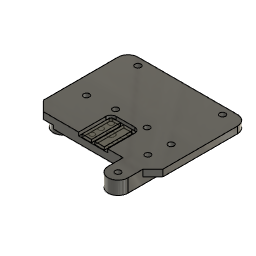
Top Plate Mjølnir (Autodesk Fusion 360 design; units mm, degrees)
Autodesk Fusion 360 part; units mm, degrees
ref_plane "WorkPlane1" through (21, -14, 35) normal (0, 0, 1) x (1, 0, 0)
sketch "Sketch2" plane through (0, 24.7, 35) normal (0, 0, 1) x (1, 0, 0)
  circle A0 centre (0, -50.925) radius 2.25
  line L0 (0, -35.7) -> (0, -50.925) construction
  line L1 (-6, -50.925) -> (6, -50.925) construction
  circle A1 centre (0, -50.925) radius 11 construction
  line L2 (18, -7.7) -> (-18, -7.7) construction
  line L3 (-30, -4.7) -> (-30, -13.7) construction
  line L4 (30, -13.7) -> (30, -4.7) construction
  circle A2 centre (-25.5, -40.2) radius 1.75 construction
  circle A3 centre (25.5, -40.2) radius 1.75 construction
  line L5 (-30, -35.7) -> (-30, -44.7) construction
  line L6 (-18, -41.7) -> (-13, -41.7) construction
  line L7 (30, -44.7) -> (30, -35.7) construction
  circle A4 centre (-25.5, -9.2) radius 1.75
  circle A5 centre (25.5, -9.2) radius 1.75
  circle A6 centre (25.5, -40.2) radius 1.75
  circle A7 centre (-25.5, -40.2) radius 1.75
  line L8 (-18, -7.7) -> (22, -7.7) construction
  line L9 (-30, -44.7) -> (-21, -44.7) construction
  line L10 (21, -44.7) -> (30, -44.7) construction
  line L11 (-30, -4.7) -> (30, -4.7)
  line L12 (30, -4.7) -> (30, -61.7)
  line L13 (30, -61.7) -> (-30, -61.7)
  line L14 (-30, -61.7) -> (-30, -4.7)
  circle A8 centre (25.5, -9.2) radius 1.75
  circle A9 centre (-25.5, -9.2) radius 1.75
  line L15 (30, -4.7) -> (21, -4.7)
  line L16 (-21, -4.7) -> (-30, -4.7)
  line L17 (-30, -13.7) -> (30, -13.7)
  line L18 (-13, -35.7) -> (-30, -35.7)
  line L19 (21, -4.7) -> (18, -7.7)
  line L20 (-18, -7.7) -> (-21, -4.7)
  line L21 (-21, -44.7) -> (-18, -41.7)
  line L22 (18, -41.7) -> (21, -44.7)
  line L23 (-30, -4.7) -> (-36, -4.7)
  line L24 (-36, -4.7) -> (-36, -61.7)
  line L25 (-36, -61.7) -> (-30, -61.7)
  line L26 (-30, -61.7) -> (-30, -4.7)
  line L27 (30, -4.7) -> (36, -4.7)
  line L28 (36, -4.7) -> (36, -61.7)
  line L29 (36, -61.7) -> (30, -61.7)
  line L30 (30, -61.7) -> (30, -4.7)
  line L31 (13, -35.7) -> (13, -41.7)
  line L32 (13, -41.7) -> (18, -41.7)
  line L33 (30, -35.7) -> (13, -35.7)
  line L34 (-13, -35.7) -> (13, -35.7)
  line L35 (-13, -41.7) -> (-13, -35.7)
  dimension "d5288" = 12
  dimension "d6330" = 4.5
  dimension "d6343" = 22
  dimension "d8089" = 10.725
  dimension "d8579" = 3.5
  dimension "d8774" = 72
  dimension "d9194" = 57
  constraint coincident A0.centre L0.end
  constraint horizontal L1
  constraint midpoint A0.centre L1
  constraint concentric A0 A1
  constraint vertical L0
  constraint coincident L2.end L8.start
  constraint concentric A4 A9
  constraint concentric A5 A8
  constraint concentric A3 A6
  constraint concentric A2 A7
  constraint equal A4 A5
  constraint equal A5 A6
  constraint equal A6 A7
  constraint horizontal L8
  constraint horizontal L11
  constraint vertical L12
  constraint horizontal L13
  constraint vertical L14
  constraint coincident L5.start L14
  constraint coincident L4.start L12
  constraint coincident L4.end L11
  constraint horizontal L23
  constraint vertical L24
  constraint horizontal L25
  constraint vertical L26
  constraint coincident L3.start L11.start
  constraint coincident L13.end L14.start
  constraint symmetric L0 L3.start L4.end
  constraint symmetric L0 L23.end L27.end
  constraint symmetric L0 L24.end L28.end
  constraint symmetric L0 L13.end L12.end
  constraint midpoint L0.start L34
  measures "d5288" distance of L1.start L1.end
  measures "d6330" diameter of A0
  measures "d6343" diameter of A1
  measures "d8089" vertical distance of A0.centre A3.centre
  measures "d8579" diameter of A4
  measures "d8774" distance of L24 L28
  measures "d9194" distance of L23.end L24.end
extrude "Extrude2" add sketch "Sketch2" along normal blind 4 makes body 1
sketch "Sketch16" plane through (0, 0, 39) normal (0, 0, 1) x (-1, 0, 0)
  circle A0 centre (0, 26.225) radius 8 construction
  line L0 (-5.6569, 20.5681) -> (5.6569, 20.5681)
  line L1 (5.6569, 20.5681) -> (5.6569, 31.8819)
  line L2 (5.6569, 31.8819) -> (-5.6569, 31.8819)
  line L3 (-5.6569, 31.8819) -> (-5.6569, 20.5681)
  line L4 (-5.6569, 20.5681) -> (5.6569, 31.8819) construction
  line L5 (5.6569, 20.5681) -> (-5.6569, 31.8819) construction
  circle A1 centre (0, 26.225) radius 2.25
  line L6 (36, 37) -> (-36, 37)
  line L7 (-36, -20) -> (36, -20)
  circle A2 centre (25.5, 15.5) radius 1.75
  circle A3 centre (25.5, -15.5) radius 1.75
  line L8 (36, -20) -> (36, 37)
  line L9 (-36, 37) -> (-36, -20)
  circle A4 centre (-25.5, -15.5) radius 1.75
  circle A5 centre (-25.5, 15.5) radius 1.75
  point P0 (0, 26.225)
  dimension "d8592" = 16
  constraint horizontal L0
  constraint perpendicular L0 L1
  constraint parallel L0 L2
  constraint parallel L1 L3
  constraint coincident A0 L0.start
  constraint coincident L4 P0
  constraint coincident L5 P0
  constraint equal L0 L3
  constraint coincident P0 A0.centre
  measures "d8592" diameter of A0
hole "Hole8" at (-5.6569, -20.5681, 39) at (-5.6569, -31.8819, 39) at (5.6569, -20.5681, 39) at (5.6569, -31.8819, 39) direction (0, 0, -1) diameter 2.9 depth 7 tip angle 118 bodies 1
hole "Hole1" at (-6, -26.225, 35) at (6, -26.225, 35) direction (0, 0, 1) diameter 2.9 depth 10 tip angle 180 bodies 1
sketch "Sketch18" plane through (0, 0, 35) normal (0, 0, -1) x (1, 0, 0)
  circle A0 centre (-25.5, -15.5) radius 1.75
  circle A1 centre (0, 26.225) radius 2.25
  circle A2 centre (-25.5, 15.5) radius 1.75
  line L0 (-36, -20) -> (36, -20)
  line L1 (36, -20) -> (36, 37)
  line L2 (36, 37) -> (-36, 37)
  line L3 (-36, 37) -> (-36, -20)
  line L4 (-19.5, 26.225) -> (17.5, 26.225) construction
  line L5 (-1, 26.225) -> (-1, 23.941) construction
  line L6 (0, 26.225) -> (0, 14.975) construction
  line L7 (0, 14.975) -> (10, 14.975) construction
  circle A3 centre (10, 14.975) radius 3
  circle A4 centre (-6, 26.225) radius 1.45
  circle A5 centre (6, 26.225) radius 1.45
  line L8 (-9.5, 24) -> (9.5, 24) construction
  line L9 (9.5, 24) -> (9.5, 14) construction
  line L10 (9.5, 14) -> (-9.5, 14) construction
  line L11 (-9.5, 14) -> (-9.5, 24) construction
  line L12 (0, 24) -> (0, 26.225) construction
  circle A6 centre (9.5, 24) radius 1.6 construction
  circle A7 centre (25.5, -15.5) radius 1.75
  circle A8 centre (25.5, 15.5) radius 1.75
  arc A9 (-13, 17) -> (13, 17) centre (0, 43.6667) ccw construction
  line L13 (13, 17) -> (13, 11) construction
  line L14 (13, 11) -> (-13, 11) construction
  circle A10 centre (5.6569, 20.5681) radius 1.45
  circle A11 centre (-5.6569, 20.5681) radius 1.45
  circle A12 centre (-5.6569, 31.8819) radius 1.45
  circle A13 centre (5.6569, 31.8819) radius 1.45
  line L15 (-13, 11) -> (-13, 17)
  point P0 (-10, 14.975)
  dimension "d8760" = 37
  dimension "d8761" = 1
  dimension "d8762" = 90
  dimension "d8763" = 10
  dimension "d8764" = 6
  dimension "d8765" = 11.25
  dimension "d8769" = 19
  dimension "d8770" = 10
  dimension "d8771" = 2.225
  dimension "d8772" = 3.2
  constraint horizontal L4
  constraint coincident A1.centre L4
  constraint midpoint L4 L5.start
  constraint perpendicular L4 L5
  constraint coincident A1.centre L6.start
  constraint perpendicular L4 L6
  constraint coincident L7.end A3.centre
  constraint symmetric L6 L7.end P0
  constraint horizontal L8
  constraint vertical L9
  constraint horizontal L10
  constraint vertical L11
  constraint midpoint L8 L12.start
  constraint perpendicular L8 L12
  constraint coincident L8.end L9.start
  measures "d8760" distance of L4.start L4.end
  measures "d8761" distance of A1.centre L5
  measures "d8762" angle of L6 L7
  measures "d8763" distance of L6.end L7.end
  measures "d8764" diameter of A3
  measures "d8765" distance of A1.centre L6.end
  measures "d8769" distance of L8.start L8.end
  measures "d8770" distance of L8.start L10.end
  measures "d8771" vertical distance of A1.centre L8.end
  measures "d8772" diameter of A6
hole "Hole11" at (9.5, -14, 35) at (-9.5, -14, 35) direction (0, 0, 1) diameter 3.4 depth 11 tip angle 118 bodies 1
chamfer "Chamfer8" distance 6 angle 45 2 edges at (-36, -37, 37) (36, -37, 37) on bodies 1
sketch "Sketch20" plane through (0, 0, 39) normal (0, 0, 1) x (-1, 0, 0)
  circle A0 centre (-9.5, 14) radius 1.7
  circle A1 centre (6, 26.225) radius 1.45
  circle A2 centre (-6, 26.225) radius 1.45
  circle A3 centre (0, 26.225) radius 2.25
  circle A4 centre (25.5, -15.5) radius 1.75
  line L0 (-36, -20) -> (36, -20)
  line L1 (36, -20) -> (36, 31)
  line L2 (30, 37) -> (-30, 37)
  line L3 (-36, 31) -> (-36, -20)
  line L4 (0, 37) -> (0, 53.2929) construction
  line L5 (-30, 37) -> (-36, 31)
  line L6 (36, 31) -> (30, 37)
  line L7 (30, 37) -> (18, 37)
  line L8 (18, 37) -> (18, 52)
  line L9 (18, 52) -> (30, 52)
  line L10 (30, 52) -> (30, 37)
  line L11 (-30, 52) -> (-30, 37)
  line L12 (-30, 37) -> (-18, 37)
  line L13 (-18, 37) -> (-18, 52)
  line L14 (-18, 52) -> (-30, 52)
  circle A5 centre (9.5, 14) radius 1.7
  circle A6 centre (-25.5, -15.5) radius 1.75
  circle A7 centre (25.5, 15.5) radius 1.75
  circle A8 centre (-25.5, 15.5) radius 1.75
  line L15 (30, 37) -> (18, 37)
  line L16 (18, 37) -> (18, 20)
  line L17 (18, 20) -> (30, 20)
  line L18 (30, 20) -> (30, 37)
  line L19 (-18, 37) -> (-18, 20)
  line L20 (-18, 20) -> (-30, 20)
  line L21 (-30, 37) -> (-18, 37)
  line L22 (-30, 20) -> (-30, 37)
  circle A9 centre (-5.6569, 20.5681) radius 1.45
  circle A10 centre (5.6569, 20.5681) radius 1.45
  circle A11 centre (5.6569, 31.8819) radius 1.45
  circle A12 centre (-5.6569, 31.8819) radius 1.45
  dimension "d9257" = 12
  dimension "d9258" = 15
  dimension "d9259" = 36
  dimension "d9371" = 17
  constraint midpoint L2 L4.start
  constraint perpendicular L2 L4
  constraint horizontal L7
  constraint vertical L8
  constraint horizontal L9
  constraint vertical L10
  constraint coincident L2.start L6.end
  constraint symmetric L4 L2.start L2.end
  constraint symmetric L4 L7.end L12.end
  constraint symmetric L4 L8.end L13.end
  constraint symmetric L4 L9.end L11.start
  constraint horizontal L15
  constraint vertical L16
  constraint horizontal L17
  constraint vertical L18
  constraint coincident L8 L7.end
  constraint symmetric L4 L16.end L19.end
  constraint symmetric L4 L17.end L20.end
  measures "d9257" distance of L2.start L7.end
  measures "d9258" distance of L2.start L9.end
  measures "d9259" distance of L8 L13
  measures "d9371" distance of L2.start L17.end
extrude "Extrude17" add sketch "Sketch20" against normal blind 8 contours L2 L11 L12 L13 L14 L21 | L2 L12 L19 L20 L21 L22 | L2 L7 L15 L16 L17 L18 bodies 1
sketch "Sketch22" plane through (0, 0, 31) normal (0, 0, -1) x (1, 0, 0)
  circle A0 centre (24, 46) radius 1.5 construction
  line L0 (24, 46) -> (24, 28) construction
  line L1 (30, 52) -> (18, 52)
  line L2 (18, 52) -> (18, 20)
  line L3 (30, 20) -> (30, 52)
  line L4 (24, 52) -> (24, 46) construction
  circle A1 centre (24, 46) radius 6
  line L5 (-30, 37) -> (-30, 20)
  line L6 (-30, 20) -> (-18, 20)
  line L7 (-18, 20) -> (-18, 37)
  line L8 (-18, 37) -> (-30, 37)
  line L9 (-30, 37) -> (-30, 20)
  line L10 (-30, 20) -> (-18, 20)
  line L11 (-18, 20) -> (-18, 37)
  line L12 (-18, 37) -> (-30, 37)
  line L13 (18, 20) -> (30, 20)
  line L14 (-18, 37) -> (18, 37)
  dimension "d9221" = 18
  dimension "d9372" = 3
  constraint coincident A0.centre L0.start
  constraint vertical L0
  constraint concentric A0 A1
  constraint tangent L3 A1
  constraint vertical L4
  constraint midpoint L1 L4.start
  constraint tangent L1 A1
  measures "d9221" distance of A0.centre L0.end
  measures "d9372" diameter of A0
fillet "Fillet9" radius 6 4 edges at (30, -52, 35) (18, -52, 35) (-18, -37, 33) (-30, -37, 33) on bodies 1
hole "Hole16" at (24, -46, 31) at (24, -28, 31) direction (0, 0, 1) diameter 3.4 depth 70 tip angle 180 bodies 1
chamfer "Chamfer9" distance 3 angle 45 2 edges at (-18, -20, 33) (18, -20, 33) on bodies 1
fillet "Fillet10" radius 6 2 edges at (36, 20, 37) (-36, 20, 37) on bodies 1
sketch "Sketch25" plane through (0, 0, 35) normal (0, 0, -1) x (1, 0, 0)
  circle A0 centre (25.5, -15.5) radius 1.75
  circle A1 centre (-25.5, -15.5) radius 1.75
  circle A2 centre (25.5, 15.5) radius 1.75
  circle A3 centre (0, 26.225) radius 2.25
  circle A4 centre (-25.5, 15.5) radius 1.75
  circle A5 centre (5.6569, 31.8819) radius 1.45
  circle A6 centre (-5.6569, 31.8819) radius 1.45
  circle A7 centre (-5.6569, 20.5681) radius 1.45
  circle A8 centre (5.6569, 20.5681) radius 1.45
  circle A9 centre (6, 26.225) radius 1.45
  circle A10 centre (-6, 26.225) radius 1.45
  circle A11 centre (-9.5, 14) radius 1.7
  circle A12 centre (9.5, 14) radius 1.7
  arc A13 (-36, -14) -> (-30, -20) centre (-30, -14) ccw
  line L0 (-30, -20) -> (30, -20)
  arc A14 (30, -20) -> (36, -14) centre (30, -14) ccw
  line L1 (36, -14) -> (36, 31)
  line L2 (36, 31) -> (30, 37)
  line L3 (30, 37) -> (30, 20)
  line L4 (30, 20) -> (21, 20)
  line L5 (21, 20) -> (18, 23)
  line L6 (18, 23) -> (18, 37)
  line L7 (18, 37) -> (-24, 37)
  arc A15 (-18, 31) -> (-24, 37) centre (-24, 31) ccw
  line L8 (-18, 31) -> (-18, 23)
  line L9 (-18, 23) -> (-21, 20)
  line L10 (-21, 20) -> (-30, 20)
  line L11 (-30, 20) -> (-30, 31)
  arc A16 (-24, 37) -> (-30, 31) centre (-24, 31) ccw
  line L12 (-24, 37) -> (-30, 37)
  line L13 (-30, 37) -> (-36, 31)
  line L14 (-36, 31) -> (-36, -14)
  arc A17 (-13, 17) -> (13, 17) centre (0, 43.6667) ccw
  line L15 (-13, 17) -> (-30, 17)
  line L16 (23.5, 17) -> (13, 17)
  line L17 (18, 17) -> (21, 20)
  line L18 (-21, 20) -> (-18, 17)
  circle A18 centre (-9.5, 14) radius 3.5
  circle A19 centre (9.5, 14) radius 3.5
  dimension "d9415" = 7
  dimension "d9416" = 7
  constraint concentric A11 A18
  constraint concentric A12 A19
  measures "d9415" diameter of A18
  measures "d9416" diameter of A19
extrude "Extrude20" add sketch "Sketch25" along normal blind 2 contours L5 L6 L7 A15 L8 L9 A17 L15 L16 L17 L18 A18 A19 bodies 1
chamfer "Chamfer10" distance 2 angle 45 3 edges at (-8.4326, -17.3333, 33) (0, -14, 33) (8.4326, -17.3333, 33) on bodies 1
sketch "Sketch26" plane through (0, 0, 39) normal (0, 0, 1) x (-1, 0, 0)
  arc A0 (30, -20) -> (36, -14) centre (30, -14) ccw
  line L0 (36, -14) -> (36, 31)
  line L1 (36, 31) -> (30, 37)
  line L2 (30, 37) -> (-18, 37)
  line L3 (-18, 37) -> (-18, 46)
  arc A1 (-18, 46) -> (-30, 46) centre (-24, 46) ccw
  line L4 (-30, 46) -> (-30, 37)
  line L5 (-30, 37) -> (-36, 31)
  line L6 (-36, 31) -> (-36, -14)
  arc A2 (-36, -14) -> (-30, -20) centre (-30, -14) ccw
  line L7 (-30, -20) -> (30, -20)
  circle A3 centre (-24, 46) radius 1.7
  circle A4 centre (-24, 28) radius 1.7
  circle A5 centre (-9.5, 14) radius 1.7
  circle A6 centre (9.5, 14) radius 1.7
  circle A7 centre (6, 26.225) radius 1.45 construction
  circle A8 centre (-6, 26.225) radius 1.45 construction
  circle A9 centre (-5.6569, 20.5681) radius 1.45 construction
  circle A10 centre (5.6569, 20.5681) radius 1.45 construction
  circle A11 centre (5.6569, 31.8819) radius 1.45 construction
  circle A12 centre (-5.6569, 31.8819) radius 1.45 construction
  circle A13 centre (25.5, 15.5) radius 1.75
  circle A14 centre (0, 26.225) radius 2.25 construction
  circle A15 centre (-25.5, 15.5) radius 1.75
  circle A16 centre (25.5, -15.5) radius 1.75
  circle A17 centre (-25.5, -15.5) radius 1.75
  line L8 (-8.725, 34.95) -> (8.725, 34.95)
  line L9 (8.725, 34.95) -> (8.725, 17.5)
  line L10 (8.725, 17.5) -> (-8.725, 17.5)
  line L11 (-8.725, 17.5) -> (-8.725, 34.95)
  line L12 (-8.725, 34.95) -> (8.725, 17.5) construction
  line L13 (8.725, 34.95) -> (-8.725, 17.5) construction
  circle A18 centre (-9.5, 14) radius 3.5
  circle A19 centre (9.5, 14) radius 3.5
  circle A20 centre (5.6569, 20.5681) radius 3.0681
  circle A21 centre (-5.6569, 20.5681) radius 3.0681
  circle A22 centre (-5.6569, 31.8819) radius 3.0681
  circle A23 centre (5.6569, 31.8819) radius 3.0681
  line L14 (8.725, 34.95) -> (-8.725, 34.95)
  line L15 (-8.725, 34.95) -> (-8.725, 37)
  line L16 (-8.725, 37) -> (8.725, 37)
  line L17 (8.725, 37) -> (8.725, 34.95)
  point P0 (0, 26.225)
  dimension "d9420" = 7
  dimension "d9421" = 7
  constraint horizontal L8
  constraint perpendicular L8 L9
  constraint parallel L8 L10
  constraint parallel L9 L11
  constraint coincident L12 P0
  constraint coincident L13 P0
  constraint coincident P0 A14.centre
  constraint concentric A5 A18
  constraint concentric A6 A19
  constraint tangent L10 A19
  constraint concentric A10 A20
  constraint tangent L10 A20
  constraint tangent L9 A20
  constraint concentric A9 A21
  constraint tangent L10 A21
  constraint concentric A12 A22
  constraint tangent L8 A22
  constraint concentric A11 A23
  constraint tangent L9 A23
  constraint horizontal L14
  constraint vertical L15
  constraint horizontal L16
  constraint vertical L17
  constraint coincident L2 L15.end
  constraint coincident L11 L8.start
  measures "d9420" diameter of A18
  measures "d9421" diameter of A19
extrude "Extrude21" cut sketch "Sketch26" against normal blind 2 contours L2 L8 L14 L15 L16 L17 | L8 L9 A23 L14 | L8 L11 A22 L14 | L8 L9 L10 L11 A20 A21 A22 A23 L14 | A23 | A22 | A20 | A21 bodies 1
sketch "Sketch27" plane through (0, 0, 37) normal (0, 0, 1) x (-1, 0, 0)
  circle A0 centre (6, 26.225) radius 1.45
  circle A1 centre (-6, 26.225) radius 1.45
  circle A2 centre (-5.6569, 20.5681) radius 1.45
  circle A3 centre (5.6569, 20.5681) radius 1.45
  circle A4 centre (5.6569, 31.8819) radius 1.45
  circle A5 centre (-5.6569, 31.8819) radius 1.45
  circle A6 centre (0, 26.225) radius 2.25
  arc A7 (5.6569, 17.5) -> (8.725, 20.5681) centre (5.6569, 20.5681) ccw
  line L0 (8.725, 20.5681) -> (8.725, 37)
  line L1 (-8.725, 37) -> (-8.725, 20.5681)
  arc A8 (-8.725, 20.5681) -> (-5.6569, 17.5) centre (-5.6569, 20.5681) ccw
  line L2 (-5.6569, 17.5) -> (5.6569, 17.5)
  line L3 (8.725, 37) -> (-8.725, 37)
extrude "Extrude22" add sketch "Sketch27" against normal blind 0.3 contours A0 | A1 | A2 | A3 | A4 | A5 | A6 bodies 1
sketch "Sketch28" plane through (0, 0, 39) normal (0, 0, 1) x (-1, 0, 0)
  line L0 (8.725, 37) -> (8.725, 20.5681)
  arc A0 (5.6569, 17.5) -> (8.725, 20.5681) centre (5.6569, 20.5681) ccw
  line L1 (5.6569, 17.5) -> (-5.6569, 17.5)
  arc A1 (-8.725, 20.5681) -> (-5.6569, 17.5) centre (-5.6569, 20.5681) ccw
  line L2 (-8.725, 20.5681) -> (-8.725, 37)
  arc A2 (30, -20) -> (36, -14) centre (30, -14) ccw
  line L3 (36, -14) -> (36, 31)
  line L4 (36, 31) -> (30, 37)
  line L5 (-8.725, 37) -> (-18, 37)
  line L6 (-18, 37) -> (-18, 46)
  arc A3 (-18, 46) -> (-30, 46) centre (-24, 46) ccw
  line L7 (-30, 46) -> (-30, 37)
  line L8 (-30, 37) -> (-36, 31)
  line L9 (-36, 31) -> (-36, -14)
  arc A4 (-36, -14) -> (-30, -20) centre (-30, -14) ccw
  line L10 (-30, -20) -> (30, -20)
  circle A5 centre (-24, 46) radius 1.7
  circle A6 centre (-24, 28) radius 1.7
  circle A7 centre (-9.5, 14) radius 1.7
  circle A8 centre (9.5, 14) radius 1.7
  circle A9 centre (25.5, 15.5) radius 1.75
  circle A10 centre (-25.5, 15.5) radius 1.75
  circle A11 centre (25.5, -15.5) radius 1.75
  circle A12 centre (-25.5, -15.5) radius 1.75
  line L11 (30, 37) -> (8.725, 37)
  line L12 (8.725, 37) -> (-8.725, 37)
  line L13 (6.725, 37) -> (6.725, 20.5681)
  arc A13 (5.6569, 19.5) -> (6.725, 20.5681) centre (5.6569, 20.5681) ccw
  line L14 (5.6569, 19.5) -> (-5.6569, 19.5)
  arc A14 (-6.725, 20.5681) -> (-5.6569, 19.5) centre (-5.6569, 20.5681) ccw
  line L15 (-6.725, 20.5681) -> (-6.725, 37)
  dimension "d9459" = 2
  constraint coincident L0.start L11.end
  constraint coincident L2.end L5.start
extrude "Extrude24" add sketch "Sketch28" against normal blind 1.7 separate body contours L12 L13 A13 L14 A14 L15 makes body 2
sketch "Sketch29" plane through (0, 0, 39) normal (0, 0, 1) x (-1, 0, 0)
  arc A0 (5.6569, 19.5) -> (6.725, 20.5681) centre (5.6569, 20.5681) ccw
  line L0 (6.725, 20.5681) -> (6.725, 37)
  line L1 (6.725, 37) -> (-6.725, 37)
  line L2 (-6.725, 37) -> (-6.725, 20.5681)
  arc A1 (-6.725, 20.5681) -> (-5.6569, 19.5) centre (-5.6569, 20.5681) ccw
  line L3 (-5.6569, 19.5) -> (5.6569, 19.5)
  line L4 (0, 19.5) -> (0, 37) construction
  line L5 (-1, 19.5) -> (1, 19.5)
  line L6 (1, 19.5) -> (1, 37)
  line L7 (1, 37) -> (-1, 37)
  line L8 (-1, 37) -> (-1, 19.5)
  line L9 (-1, 19.5) -> (1, 37) construction
  line L10 (1, 19.5) -> (-1, 37) construction
  point P0 (0, 28.25)
  dimension "d9462" = 2
  constraint midpoint L3 L4.start
  constraint midpoint L1 L4.end
  constraint horizontal L5
  constraint perpendicular L5 L6
  constraint parallel L5 L7
  constraint parallel L6 L8
  constraint coincident L3 L5.start
  constraint coincident L9 P0
  constraint coincident L10 P0
  constraint midpoint L4 P0
  measures "d9462" distance of L6.end L7.end
extrude "Extrude25" cut sketch "Sketch29" against normal blind 2 contours L1 L3 L5 L6 L7 L8 bodies 2 makes body 3 at (2.9083, -25.6894, 39)
sketch "Sketch24" plane through (0, 0, 31) normal (0, 0, -1) x (1, 0, 0)
  line L0 (18, 46) -> (18, 23)
  line L1 (21, 20) -> (30, 20)
  line L2 (30, 20) -> (30, 46)
  circle A0 centre (24, 46) radius 1.7
  circle A1 centre (24, 28) radius 1.7
  arc A2 (30, 46) -> (18, 46) centre (24, 46) ccw
  line L3 (18, 23) -> (21, 20)
equation "d5284 = Part_Thickness"
equation "d8089 = hotend_offset"
equation "Part_Thickness = 4 mm" comment "Thickness of Printed Parts"
equation "hotend_offset = 13.725 mm - 3 mm" comment "Hotend Offset From Carrier"
